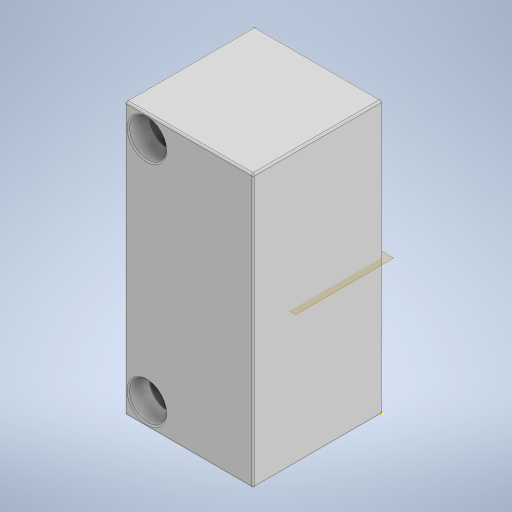
# Autodesk Inventor part: springHolder
Saved by Autodesk Inventor 2023 (Build 270158000, 158)
## iProperties
Created: 2023-03-06
Part Number: springHolder
Material: Generic
Document SubType Name: Modeling
Designer: gorki
Density: 1 g/cm^3
Appearance: Default
Author: gorki
Autodesk Inventor part; units mm, degrees
ref_plane "YZ Plane" through (0, 0, 0) normal (1, 0, 0) x (0, 1, 0)
ref_plane "XZ Plane" through (0, 0, 0) normal (0, 1, 0) x (-1, 0, 0)
ref_plane "XY Plane" through (0, 0, 0) normal (0, 0, 1) x (1, 0, 0)
sketch "Sketch5" plane through (0, 0, 0) normal (0, 0, 1) x (1, 0, 0)
  line L0 (0, 0) -> (-34.6, 0)
  line L1 (-34.6, 0) -> (-34.6, 73.3)
  line L2 (-34.6, 73.3) -> (0, 73.3)
  line L3 (0, 73.3) -> (0, 0)
  dimension "d7" = 34.6
  dimension "d8" = 73.3
  constraints: 8 end point, 2 parallel, 1 horizontal, 1 perpendicular
  measures "d7" distance of L1.end L2.end
  measures "d8" distance of L0.end L1.end
sketch "Sketch6" plane through (0, 0, 0) normal (0, 0, 1) x (1, 0, 0)
  point P0 (0, 0)
extrude "Extrusion3" add sketch "Sketch5" along normal blind 35
sketch "Sketch7" plane through (0, 0, 35) normal (0, 0, 1) x (1, 0, 0)
  line L0 (-34.6, 0) -> (0, 0) projected
  line L1 (-34.6, 0) -> (-34.6, 6)
  line L2 (-34.6, 73.3) -> (-34.6, 0) projected
  line L3 (-34.6, 6) -> (-28.6, 6)
  dimension "d11" = 6
  dimension "d12" = 6
  constraints: 4 end point, 1 perpendicular, 1 point on line
  measures "d11" distance of L0.start L1.end
  measures "d12" distance of L1.end L3.end
hole "Hole1" at (-28.6, 6, 35) direction (0, 0, -1) diameter 5.3 end through all counterbore diameter 10 counterbore depth 5.7 clearance for "Socket Head Cap Screw ISO 4762" size "M5" standard "ISO"
ref_plane "Work Plane1" through (-34.6, 36.65, 0) normal (0, 1, 0) x (1, 0, 0)
mirror "Mirror1" about plane through (-34.6, 36.65, 0) normal (0, 1, 0) of "Hole1"
sketch "Sketch8" plane through (-34.6, 0, 0) normal (-1, 0, 0) x (0, 0, 1)
  point P0 (0, 0)
sketch "Sketch9" plane through (-34.6, 0, 0) normal (-1, 0, 0) x (0, 0, 1)
  line L0 (0, 0) -> (35, 0) projected
  line L1 (0, 0) -> (0, 36.65)
  line L2 (0, 73.3) -> (0, 0) projected
  line L3 (0, 36.65) -> (27.5, 36.65)
  circle A0 centre (27.5, 36.65) radius 4.5
  dimension "d20" = 36.65
  dimension "d21" = 27.5
  dimension "d22" = 9
  constraints: 4 end point, 1 centre point, 1 coincident, 1 midpoint, 1 perpendicular
  measures "d20" distance of L0.start L1.end
  measures "d21" distance of L1.end L3.end
  measures "d22" diameter of A0
extrude "Extrusion4" cut sketch "Sketch9" against normal blind 5
fillet "Fillet1" radius 0.5 12 edges at (0, 73.3, 17.5) (-34.6, 73.3, 17.5) (0, 0, 17.5) (-34.6, 0, 17.5) (-17.3, 0, 35) (-17.3, 0, 0) (0, 36.65, 0) (-34.6, 36.65, 0) (-17.3, 73.3, 0) (-17.3, 73.3, 35) (0, 36.65, 35) (-34.6, 36.65, 35)
chamfer "Chamfer1" distance 0.35 angle 45 1 edges at (-28.6, 11, 35)
chamfer "Chamfer2" distance 0.35 angle 45 1 edges at (-28.6, 62.3, 35)
chamfer "Chamfer3" distance 0.35 angle 45 2 edges at (-28.6, 8.65, 0) (-28.6, 64.65, 0)
chamfer "Chamfer4" distance 0.35 angle 45 1 edges at (-34.6, 36.65, 23)
body "Solid2"
